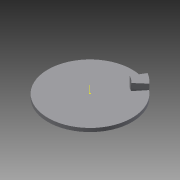
# Autodesk Inventor part: male bayonet connector 10
Saved by Autodesk Inventor 2015 (Build 190159000, 159)
## iProperties
Created: 2014-06-11
Part Number: male bayonet connector 10
Material: Generic
Document SubType Name: Modeling
Designer: ericd_000
Density: 1 g/cm^3
Appearance: Default
Author: ericd_000
Autodesk Inventor part; units mm, degrees
ref_plane "YZ Plane" through (0, 0, 0) normal (1, 0, 0) x (0, 1, 0)
ref_plane "XZ Plane" through (0, 0, 0) normal (0, 1, 0) x (-1, 0, 0)
ref_plane "XY Plane" through (0, 0, 0) normal (0, 0, 1) x (1, 0, 0)
sketch "Sketch19" plane through (0, 0, 0) normal (0, 0, 1) x (1, 0, 0)
  circle A0 centre (0, 0) radius 59
  dimension "d94" = 118
  constraints: 1 centre point, 1 coincident
  measures "d94" diameter of A0
extrude "Extrusion20" add sketch "Sketch19" along normal blind 5
sketch "Sketch21" plane through (0, 0, 5) normal (0, 0, 1) x (1, 0, 0)
  point P0 (0, 0)
sketch "Sketch23" plane through (0, 0, 5) normal (0, 0, 1) x (1, 0, 0)
  line L0 (0, 0) -> (30.298, 50.6264) construction
  circle A0 centre (0, 0) radius 59 construction
  line L1 (0, 0) -> (37.049, 45.917) construction
  circle A1 centre (0, 0) radius 59 construction
  line L2 (37.049, 45.917) -> (25.7528, 31.917)
  line L3 (25.7528, 31.917) -> (20.8552, 34.848)
  line L4 (20.8552, 34.848) -> (30.298, 50.6264)
  arc A2 (37.049, 45.917) -> (30.298, 50.6264) centre (0, 0) ccw
  dimension "d105" = 172
  dimension "d106" = 14
  constraints: 10 end point, 2 collinear, 2 point on circle, 1 centre point, 1 perpendicular, 5 other
  measures "d105" angle of L0 L1
  measures "d106" vertical distance of L1.end L2.end
extrude "Extrusion21" add sketch "Sketch23" along normal blind 15
sketch "Sketch24" plane through (37.049, 45.917, 20) normal (0.7782548, -0.6279487, 0) x (0, 0, -1)
  line L0 (0, 0) -> (7, 0)
  line L1 (15, 0) -> (0, 0) projected
  line L2 (15, -17.989) -> (0, -17.989) projected
  line L3 (7, -17.989) -> (0, -17.989)
  line L4 (0, -17.989) -> (0, 0)
  line L5 (15, -0.5742) -> (0, -0.5742) projected
  line L6 (7, 0) -> (7, -17.989)
  line L7 (24, -59) -> (-4, -59) projected
  point P0 (20, -59)
  dimension "d109" = 7
  dimension "d110" = 7
  constraints: 8 end point, 2 point on line, 1 collinear, 1 perpendicular
  measures "d109" distance of L0.start L0.end
  measures "d110" distance of L3.start L2.end
revolve "Revolution1" add sketch "Sketch24" angle 10 about axis through (0, 0, 5) along (0, 0, -1)
body "Solid2"
